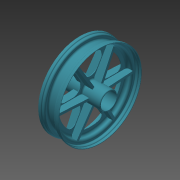
# Autodesk Inventor part: Obręcz_koła_przedniego
Saved by Autodesk Inventor 2015 (Build 190159000, 159)
## iProperties
Created: 2015-11-29
Part Number: Obręcz_koła_przedniego
Material: Aluminium 6061
Document SubType Name: Modeling
Designer: graaapsik
Density: 2.71 g/cm^3
Appearance: Niebieska z odcieniem szarości
Author: graaapsik
Autodesk Inventor part; units mm, degrees
ref_plane "YZ Plane" through (0, 0, 0) normal (1, 0, 0) x (0, 1, 0)
ref_plane "XY Plane" through (0, 0, 0) normal (0, 0, 1) x (1, 0, 0)
sketch "Szkic1" plane through (0, 0, 0) normal (0, 0, 1) x (1, 0, 0)
  line L0 (0, 6.7879) -> (0, 0) construction
  line L1 (0, 0) -> (7.1213, 0) construction
  line L2 (-21, 10.75) -> (-2.375, 10.75)
  arc A0 (-2.375, 10.75) -> (-0.375, 12.75) centre (-2.375, 12.75) ccw
  line L3 (-0.375, 12.75) -> (-0.375, 42)
  arc A1 (-0.375, 42) -> (-3.375, 45) centre (-3.375, 42) ccw
  line L4 (-3.375, 45.7) -> (0, 45.7)
  arc A2 (-21, 10.75) -> (-22, 9.75) centre (-21, 9.75) ccw
  line L5 (-22, 9.75) -> (-22, 0)
  line L6 (-5.375, 47.7) -> (-5.375, 48.7)
  line L7 (-6.875, 50.2) -> (-8.5, 50.2)
  line L8 (-8.883, 50.3786) -> (-9.1796, 50.7321)
  line L9 (-9.7542, 51) -> (-12.35, 51)
  line L10 (-12.35, 50.3) -> (-9.7542, 50.3)
  line L11 (-9.7159, 50.2821) -> (-9.4193, 49.9287)
  line L12 (-8.5, 49.5) -> (-6.875, 49.5)
  line L13 (-6.075, 48.7) -> (-6.075, 47.7)
  arc A3 (-5.375, 47.7) -> (-3.375, 45.7) centre (-3.375, 47.7) ccw
  arc A4 (-5.375, 48.7) -> (-6.875, 50.2) centre (-6.875, 48.7) ccw
  arc A5 (-9.1796, 50.7321) -> (-9.7542, 51) centre (-9.7542, 50.25) ccw
  arc A6 (-9.7159, 50.2821) -> (-9.7542, 50.3) centre (-9.7542, 50.25) ccw
  arc A7 (-8.883, 50.3786) -> (-8.5, 50.2) centre (-8.5, 50.7) ccw
  arc A8 (-9.4193, 49.9287) -> (-8.5, 49.5) centre (-8.5, 50.7) ccw
  arc A9 (-6.075, 48.7) -> (-6.875, 49.5) centre (-6.875, 48.7) ccw
  arc A10 (-6.075, 47.7) -> (-3.375, 45) centre (-3.375, 47.7) ccw
  line L14 (-12.5, 50.85) -> (-12.5, 50.45)
  arc A11 (-12.35, 51) -> (-12.5, 50.85) centre (-12.35, 50.85) ccw
  arc A12 (-12.5, 50.45) -> (-12.35, 50.3) centre (-12.35, 50.45) ccw
  line L15 (-8.5, 50.2) -> (-8.5, 51.6952) construction
  line L16 (-22, 0) -> (0, 0)
  line L17 (21, 10.75) -> (2.375, 10.75)
  arc A13 (0.375, 12.75) -> (2.375, 10.75) centre (2.375, 12.75) ccw
  line L18 (0.375, 12.75) -> (0.375, 42)
  arc A14 (3.375, 45) -> (0.375, 42) centre (3.375, 42) ccw
  line L19 (3.375, 45.7) -> (0, 45.7)
  arc A15 (22, 9.75) -> (21, 10.75) centre (21, 9.75) ccw
  line L20 (22, 9.75) -> (22, 0)
  line L21 (5.375, 47.7) -> (5.375, 48.7)
  line L22 (6.875, 50.2) -> (8.5, 50.2)
  line L23 (8.883, 50.3786) -> (9.1796, 50.7321)
  line L24 (9.7542, 51) -> (12.35, 51)
  line L25 (12.35, 50.3) -> (9.7542, 50.3)
  line L26 (9.7159, 50.2821) -> (9.4193, 49.9287)
  line L27 (8.5, 49.5) -> (6.875, 49.5)
  line L28 (6.075, 48.7) -> (6.075, 47.7)
  arc A16 (3.375, 45.7) -> (5.375, 47.7) centre (3.375, 47.7) ccw
  arc A17 (6.875, 50.2) -> (5.375, 48.7) centre (6.875, 48.7) ccw
  arc A18 (9.7542, 51) -> (9.1796, 50.7321) centre (9.7542, 50.25) ccw
  arc A19 (9.7542, 50.3) -> (9.7159, 50.2821) centre (9.7542, 50.25) ccw
  arc A20 (8.5, 50.2) -> (8.883, 50.3786) centre (8.5, 50.7) ccw
  arc A21 (8.5, 49.5) -> (9.4193, 49.9287) centre (8.5, 50.7) ccw
  arc A22 (6.875, 49.5) -> (6.075, 48.7) centre (6.875, 48.7) ccw
  arc A23 (3.375, 45) -> (6.075, 47.7) centre (3.375, 47.7) ccw
  line L29 (12.5, 50.85) -> (12.5, 50.45)
  arc A24 (12.5, 50.85) -> (12.35, 51) centre (12.35, 50.85) ccw
  arc A25 (12.35, 50.3) -> (12.5, 50.45) centre (12.35, 50.45) ccw
  line L30 (8.5, 50.2) -> (8.5, 51.6952) construction
  line L31 (22, 0) -> (0, 0)
  point P0 (-6.075, 45)
  point P1 (-5.375, 45.7)
  point P2 (3.375, 45.7)
  point P3 (6.075, 45)
  point P4 (5.375, 45.7)
  dimension "d102" = 0.7
  dimension "d103" = 0.7
  dimension "d104" = 0.7
  dimension "d105" = 0.7
  dimension "d106" = 0.7
  dimension "d107" = 0.15
  dimension "d108" = 6
  dimension "d111" = 2
  dimension "d112" = 0.7
  dimension "d115" = 0.7
  dimension "d116" = 0.7
  dimension "d117" = 0.7
  dimension "d118" = 1.5
  dimension "d119" = 0.5
  dimension "d120" = 0.75
  dimension "d121" = 40
  dimension "d124" = 4.5
  dimension "d131" = 12.5
  dimension "d132" = 22
  dimension "d133" = 10.75
  dimension "d134" = 1
  dimension "d135" = 2
  dimension "d136" = 0.375
  dimension "d137" = 51
  dimension "d138" = 3
  dimension "d139" = 4
  constraints: 64 end point, 54 point on circle, 44 symmetric about line, 26 centre point, 24 tangent, 7 point on line, 6 parallel, 4 perpendicular, 3 vertical, 1 equal radius, 23 other
  measures "d103" distance between parallel lines of L13 L6
  measures "d104" distance between parallel lines of L7 L12
  measures "d105" distance between parallel lines of L8 L11
  measures "d106" distance between parallel lines of L9 L10
  measures "d107" radius of A11
  measures "d111" radius of A3
  measures "d112" radial gap between concentric circles of A10 A3
  measures "d115" radial gap between concentric circles of A4 A9
  measures "d116" radial gap between concentric circles of A7 A8
  measures "d117" radial gap between concentric circles of A5 A6
  measures "d118" radius of A4
  measures "d119" radius of A7
  measures "d120" radius of A5
  measures "d121" angle of L15 L8
  measures "d124" distance from line of A1.end L12
  measures "d131" distance between parallel lines of L0 L14
  measures "d132" distance between parallel lines of L0 L5
  measures "d133" distance between parallel lines of L16 L2
  measures "d134" radius of A2
  measures "d135" radius of A0
  measures "d136" distance between parallel lines of L0 L3
  measures "d137" distance between parallel lines of L9 L16
  measures "d138" radius of A1
  measures "d139" distance from line of L7.end L14
revolve "Obrót1" add sketch "Szkic1" angle 360 about axis through (0, 0, 0) along (1, 0, 0)
sketch "Szkic2" plane through (22, 0, 0) normal (1, 0, 0) x (0, 0, -1)
  circle A0 centre (0, 0) radius 9.75
  circle A1 centre (0, 0) radius 9.75 projected
  constraints: 1 centre point, 1 coincident
hole "Otwór na oś" at (22, 0, 0) direction (-1, 0, 0) diameter 19.5 end through all
sketch "Szkic5" plane through (0.375, 0, 0) normal (1, 0, 0) x (0, 0, -1)
  circle A0 centre (0, 0) radius 42
  line L0 (0, 0) -> (0, 51.199) construction
  line L1 (0, 0) -> (42.2342, 24.3839) construction
  line L2 (2.5, 31.7313) -> (2.5, 21.6506)
  line L3 (17.5, 12.9904) -> (26.2301, 18.0307)
  arc A1 (27.473, 27.4692) -> (10.0525, 37.5269) centre (0, 0) ccw
  arc A2 (10.0525, 37.5269) -> (2.5, 31.7313) centre (8.5, 31.7313) ccw
  arc A3 (26.2301, 18.0307) -> (27.473, 27.4692) centre (23.2301, 23.2268) ccw
  circle A4 centre (0, 0) radius 50.85
  arc A5 (2.5, 21.6506) -> (17.5, 12.9904) centre (12.5, 21.6506) ccw
  circle A6 centre (0, 0) radius 42 projected
  circle A7 centre (0, 0) radius 12.75 projected
  point P0 (2.5, -38.7695)
  point P1 (-34.8254, -17.2197)
  dimension "d56" = 60
  dimension "d57" = 2.5
  dimension "d58" = 2.5
  dimension "d59" = 6
  dimension "d61" = 10
  dimension "d62" = 12
  constraints: 10 point on circle, 8 end point, 6 centre point, 6 tangent, 2 parallel, 2 point on line, 1 concentric, 1 equal radius, 1 vertical
  measures "d56" angle of L1 L0
  measures "d57" distance between parallel lines of L0 L2
  measures "d58" distance between parallel lines of L1 L3
  measures "d59" radius of A2
  measures "d61" radius of A5
  measures "d62" radial gap between concentric circles of A4 A1
extrude "Wyciągnięcie zmniejszenie masy" cut sketch "Szkic5" against normal up to next contours A2 A1 A3 L3 A5 L2
ref_plane "Płaszczyzna konstrukcyjna1" through (0, 45, 0) normal (0, 1, 0) x (-1, 0, 0)
sketch "Szkic6" plane through (0, 45, 0) normal (0, 1, 0) x (-1, 0, 0)
  line L0 (-7.5, 1.5) -> (7.5, 1.5)
  line L1 (7.5, 1.5) -> (7.5, -1.5)
  line L2 (7.5, -1.5) -> (-7.5, -1.5)
  line L3 (-7.5, -1.5) -> (-7.5, 1.5)
  line L4 (-7.5, 1.5) -> (7.5, -1.5) construction
  line L5 (7.5, 1.5) -> (-7.5, -1.5) construction
  point P0 (0, 0)
  dimension "d69" = 15
  dimension "d70" = 3
  constraints: 12 end point, 2 midpoint, 2 parallel, 1 horizontal, 1 perpendicular
  measures "d69" distance of L0.start L0.end
  measures "d70" distance of L0.end L1.end
sketch "Szkic8" plane through (0, 0, 0) normal (0, 1, 0) x (-1, 0, 0)
  line L0 (-10.25, 1.5) -> (10.25, 1.5) projected
  line L1 (10.25, -1.5) -> (-10.25, -1.5) projected
  line L2 (10.25, 1.5) -> (10.25, -1.5) projected
  line L3 (-10.25, -1.5) -> (-10.25, 1.5) projected
  point P0 (0, 0)
loft "Wyciągnięcie wzmocnienie" add profiles "Szkic8", "Szkic6"
sketch "Szkic9" plane through (-10.25, 0, 1.5) normal (0, -1, 0) x (1, 0, 0)
  line L0 (20.5, 0) -> (0, 0) projected
  line L1 (0, 0) -> (0, -3) projected
  line L2 (0, -3) -> (20.5, -3) projected
  line L3 (20.5, -3) -> (20.5, 0) projected
  point P0 (10.25, -1.5)
extrude "Wyciągnięcie proste2" cut sketch "Szkic9" against normal up to surface round surface about axis through (-128.8111, 0, 0) along (1, 0, 0) radius 9.75 far side no
pattern_circular "Szyk wzmocnień" count 6 over 360 about axis through (1.6875, 0, 0) along (1, 0, 0) of "Wyciągnięcie zmniejszenie masy", "Wyciągnięcie wzmocnienie", "Wyciągnięcie proste2"
ref_plane "Płaszczyzna konstrukcyjna3" through (0, 22.5, 38.9711) normal (0, 0.5, 0.8660254) x (-1, 0, 0)
ref_plane "Płaszczyzna konstrukcyjna4" through (0, -22.5, 38.9711) normal (0, -0.5, 0.8660254) x (-1, 0, 0)
ref_plane "Płaszczyzna konstrukcyjna5" through (0, -45, 0) normal (0, -1, 0) x (-1, 0, 0)
ref_plane "Płaszczyzna konstrukcyjna6" through (0, -22.5, -38.9711) normal (0, -0.5, -0.8660254) x (-1, 0, 0)
ref_plane "Płaszczyzna konstrukcyjna7" through (0, 22.5, -38.9711) normal (0, 0.5, -0.8660254) x (-1, 0, 0)
